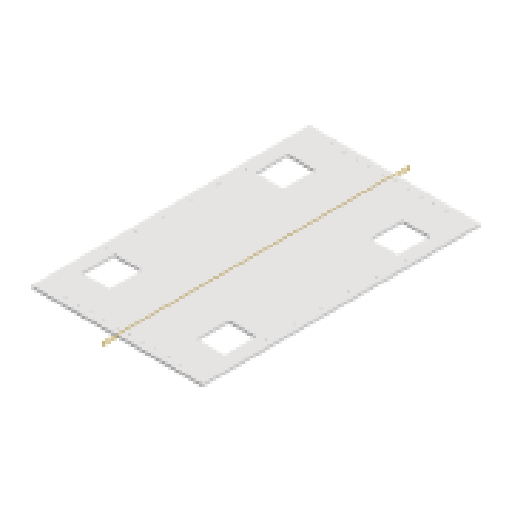
# Autodesk Inventor part: platform
Saved by Autodesk Inventor 2023.2 (Build 272271030, 271C)
## iProperties
Created: 2024-10-30
Part Number: platform
Material: Типовые
Document SubType Name: Modeling
Designer: I9232
Density: 1 g/cm^3
Appearance: По умолчанию
Author: I9232
Autodesk Inventor part; units mm, degrees
ref_plane "XZ Plane" through (0, 0, 0) normal (0, 1, 0) x (-1, 0, 0)
ref_plane "XY Plane" through (0, 0, 0) normal (0, 0, 1) x (1, 0, 0)
sketch "Эскиз1" plane through (0, 0, 0) normal (0, 1, 0) x (-1, 0, 0)
  line L0 (200, 325) -> (-200, 325)
  line L1 (-200, 325) -> (-200, -325)
  line L2 (-200, -325) -> (200, -325)
  line L3 (200, -325) -> (200, 325)
  line L4 (200, 325) -> (-200, -325) construction
  line L5 (-200, 325) -> (200, -325) construction
  point P0 (0, 0)
  dimension "d0" = 650
  dimension "d1" = 400
  constraints: 12 end point, 2 midpoint, 2 parallel, 1 horizontal, 1 perpendicular
  measures "d0" distance of L0.end L1.end
  measures "d1" distance of L1.end L2.end
extrude "Выдавливание1" add sketch "Эскиз1" along normal mid plane 6
fillet "Сопряжение1" radius 4 4 edges at (-200, 0, -325) (200, 0, -325) (200, 0, 325) (-200, 0, 325)
sketch "Эскиз3" plane through (0, 3, 0) normal (0, 1, 0) x (1, 0, 0)
  circle A0 centre (185, -137.5) radius 2
  arc A1 (-200, -321) -> (-196, -325) centre (-196, -321) ccw projected
  line L0 (-196, -325) -> (196, -325) projected
  arc A2 (196, -325) -> (200, -321) centre (196, -321) ccw projected
  line L1 (200, -321) -> (200, 321) projected
  arc A3 (200, 321) -> (196, 325) centre (196, 321) ccw projected
  line L2 (196, 325) -> (-196, 325) projected
  arc A4 (-196, 325) -> (-200, 321) centre (-196, 321) ccw projected
  line L3 (-200, 321) -> (-200, -321) projected
  line L4 (185, -413) -> (185, 413)
  circle A5 centre (185, -82.5) radius 2
  line L5 (185, -358) -> (185, 468)
  circle A6 centre (185, -27.5) radius 2
  line L6 (185, -303) -> (185, 523)
  circle A7 centre (185, 27.5) radius 2
  line L7 (185, -248) -> (185, 578)
  circle A8 centre (185, 82.5) radius 2
  line L8 (185, -193) -> (185, 633)
  circle A9 centre (185, 137.5) radius 2
  line L9 (185, -138) -> (185, 688)
  line L10 (0, -413) -> (0, 413) construction
  circle A10 centre (-185, -137.5) radius 2
  circle A11 centre (-185, -82.5) radius 2
  circle A12 centre (-185, -27.5) radius 2
  circle A13 centre (-185, 27.5) radius 2
  circle A14 centre (-185, 82.5) radius 2
  circle A15 centre (-185, 137.5) radius 2
  line L11 (-130.8, 310) -> (-209.2, 310) construction
  circle A16 centre (-135, 310) radius 2
  circle A17 centre (-105, 310) radius 2
  circle A18 centre (-75, 310) radius 2
  circle A19 centre (-45, 310) radius 2
  circle A20 centre (-15, 310) radius 2
  circle A21 centre (15, 310) radius 2
  circle A22 centre (45, 310) radius 2
  circle A23 centre (75, 310) radius 2
  circle A24 centre (105, 310) radius 2
  circle A25 centre (135, 310) radius 2
  line L12 (280, 0) -> (-280, 0) construction
  circle A26 centre (-135, -310) radius 2
  circle A27 centre (-105, -310) radius 2
  circle A28 centre (-75, -310) radius 2
  circle A29 centre (-45, -310) radius 2
  circle A30 centre (-15, -310) radius 2
  circle A31 centre (15, -310) radius 2
  circle A32 centre (45, -310) radius 2
  circle A33 centre (75, -310) radius 2
  circle A34 centre (105, -310) radius 2
  circle A35 centre (135, -310) radius 2
  point P0 (0, 0)
  point P1 (-130.8, -310)
  point P2 (185, 325)
  point P3 (185, 139.5)
  point P4 (185, 135.5)
  point P5 (185, 84.5)
  point P6 (185, 80.5)
  point P7 (185, 29.5)
  point P8 (185, 25.5)
  point P9 (185, -25.5)
  point P10 (185, -29.5)
  point P11 (185, -80.5)
  point P12 (185, -84.5)
  point P13 (185, -135.5)
  point P14 (185, -139.5)
  point P15 (185, -325)
  dimension "d7" = 4
  dimension "d10" = 55
  dimension "d15" = 4
  dimension "d16" = 65
  dimension "d17" = 187.5
  dimension "d20" = 30
  constraints: 32 centre point, 18 end point, 17 symmetric about line, 7 point on line, 3 horizontal, 3 vertical, 1 collinear, 66 other
  measures "d7" diameter of A0
  measures "d10" distance of A0.centre A5.centre
  measures "d15" diameter of A16
  measures "d16" distance from line of L3 A16.centre
  measures "d17" distance from line of L0 A0.centre
  measures "d20" distance of A16.centre A17.centre
extrude "Выдавливание3" cut sketch "Эскиз3" against normal up to surface (6 mm away) contours A0 L4 | L4 A0 | A5 L4 | L4 A5 | A6 L4 | L4 A6 | A7 L4 | L4 A7 | A8 L4 | L4 A8 | A9 L4 | L4 A9 | A10 | A11 | A12 | A13 | A14 | A15 | A16 | A17 | A18 | A19 | A20 | A21 | A22 | A23 | A24 | A25 | A26 | A27 | A28 | A29 | A30 | A31 | A32 | A33 | A34 | A35
sketch "Эскиз4" plane through (0, -3, 0) normal (0, -1, 0) x (1, 0, 0)
  line L0 (-200, 162.6052) -> (-135, 162.6052)
  line L1 (-135, 162.6052) -> (-135, 237.6052)
  line L2 (-135, 237.6052) -> (-200, 237.6052)
  line L3 (-200, 237.6052) -> (-200, 162.6052)
  line L4 (-200, 0) -> (200, 0) construction
  line L5 (0, 455) -> (0, -455) construction
  line L6 (-135, -162.6052) -> (-135, -237.6052)
  line L7 (-200, -237.6052) -> (-200, -162.6052)
  line L8 (200, 162.6052) -> (135, 162.6052)
  line L9 (135, 162.6052) -> (135, 237.6052)
  line L10 (135, 237.6052) -> (200, 237.6052)
  line L11 (200, 237.6052) -> (200, 162.6052)
  line L12 (200, -237.6052) -> (200, -162.6052)
  line L13 (200, -162.6052) -> (135, -162.6052)
  line L14 (135, -162.6052) -> (135, -237.6052)
  line L15 (135, -237.6052) -> (200, -237.6052)
  line L16 (-200, -237.6052) -> (-135, -237.6052)
  line L17 (-135, -162.6052) -> (-200, -162.6052)
  line L18 (-151.5046, 223.8552) -> (-192.0046, 223.8552) projected
  line L19 (-200, 321) -> (-200, -321) projected
  point P0 (0, 0)
  dimension "d27" = 75
  dimension "d28" = 65
  dimension "d33" = 13.75
  constraints: 32 end point, 12 symmetric about line, 2 horizontal, 2 parallel, 2 perpendicular, 1 point on line
  measures "d27" distance of L0.end L1.end
  measures "d28" distance of L1.end L2.end
  measures "d33" distance between parallel lines of L2 L18
extrude "Выдавливание4" cut sketch "Эскиз4" against normal up to surface (6 mm away)
fillet "Сопряжение2" radius 5 14 edges at (200, 0, -237.6052) (135, 0, -237.6052) (135, 0, -162.6052) (200, 0, -162.6052) (135, 0, 162.6052) (135, 0, 237.6052) (200, 0, 237.6052) (200, 0, 162.6052) (-200, 0, 237.6052) (-200, 0, 162.6052) (-135, 0, 162.6052) (-135, 0, 237.6052) (-135, 0, -162.6052) (-135, 0, -237.6052)
